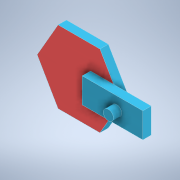
# Autodesk Inventor part: base
Saved by Autodesk Inventor 2021 (Build 250183000, 183)
## iProperties
Created: 2021-08-13
Part Number: base
Material: Genérico
Document SubType Name: Modeling
Designer: uriel
Density: 1 g/cm^3
Appearance: Turquesa
Author: uriel
Autodesk Inventor part; units mm, degrees
ref_plane "YZ Plane" through (0, 0, 0) normal (1, 0, 0) x (0, 1, 0)
ref_plane "XZ Plane" through (0, 0, 0) normal (0, 1, 0) x (-1, 0, 0)
ref_plane "XY Plane" through (0, 0, 0) normal (0, 0, 1) x (1, 0, 0)
sketch "Boceto1" plane through (0, 0, 0) normal (0, 0, 1) x (1, 0, 0)
  line L0 (50, 0) -> (25, -43.3013)
  line L1 (25, -43.3013) -> (-25, -43.3013)
  line L2 (-25, -43.3013) -> (-50, 0)
  line L3 (-50, 0) -> (-25, 43.3013)
  line L4 (-25, 43.3013) -> (25, 43.3013)
  line L5 (25, 43.3013) -> (50, 0)
  point P0 (0, 0)
  point P1 (0, 0)
  dimension "d3" = 50
  constraints: 12 end point, 1 coincident, 13 other
  measures "d3" distance of L4.end L0.start
extrude "Extrusión1" add sketch "Boceto1" along normal blind 10
sketch "Boceto2" plane through (0, 0, 10) normal (0, 0, 1) x (1, 0, 0)
  line L0 (13.773, -15) -> (86.227, -15)
  line L1 (86.227, -15) -> (86.227, 15)
  line L2 (86.227, 15) -> (13.773, 15)
  line L3 (13.773, 15) -> (13.773, -15)
  line L4 (25, -43.3013) -> (50, 0) projected
  line L5 (13.773, -15) -> (86.227, 15) construction
  line L6 (86.227, -15) -> (13.773, 15) construction
  dimension "d7" = 30
  dimension "d8" = 72.454
  constraints: 12 end point, 2 midpoint, 2 parallel, 1 horizontal, 1 perpendicular
  measures "d7" distance of L1.end L0.end
  measures "d8" distance of L1.end L2.end
extrude "Extrusión2" add sketch "Boceto2" along normal blind 10
sketch "Boceto3" plane through (0, 0, 20) normal (0, 0, 1) x (1, 0, 0)
  line L0 (13.773, 15) -> (41.3397, 15) projected
  line L1 (41.3397, 15) -> (25, 43.3013) projected
  line L2 (25, 43.3013) -> (-25, 43.3013) projected
  line L3 (-25, 43.3013) -> (-50, 0) projected
  line L4 (-50, 0) -> (-25, -43.3013) projected
  line L5 (-25, -43.3013) -> (25, -43.3013) projected
  line L6 (25, -43.3013) -> (41.3397, -15) projected
  line L7 (41.3397, -15) -> (13.773, -15) projected
  line L8 (13.773, -15) -> (13.773, 15) projected
  line L9 (0, 0) -> (55, 0)
  circle A0 centre (55, 0) radius 6
  line L10 (13.773, 15) -> (41.3397, 15) projected
  line L11 (41.3397, 15) -> (25, 43.3013) projected
  line L12 (25, 43.3013) -> (-25, 43.3013) projected
  line L13 (-25, 43.3013) -> (-50, 0) projected
  line L14 (-50, 0) -> (-25, -43.3013) projected
  line L15 (-25, -43.3013) -> (25, -43.3013) projected
  line L16 (25, -43.3013) -> (41.3397, -15) projected
  line L17 (41.3397, -15) -> (13.773, -15) projected
  line L18 (13.773, -15) -> (13.773, 15) projected
  line L19 (13.773, 15) -> (41.3397, 15) projected
  line L20 (41.3397, 15) -> (25, 43.3013) projected
  line L21 (25, 43.3013) -> (-25, 43.3013) projected
  line L22 (-25, 43.3013) -> (-50, 0) projected
  line L23 (-50, 0) -> (-25, -43.3013) projected
  line L24 (-25, -43.3013) -> (25, -43.3013) projected
  line L25 (25, -43.3013) -> (41.3397, -15) projected
  line L26 (41.3397, -15) -> (13.773, -15) projected
  line L27 (13.773, -15) -> (13.773, 15) projected
  line L28 (86.227, 15) -> (13.773, 15) projected
  dimension "d9" = 55
  dimension "d10" = 12
  constraints: 2 end point, 1 centre point, 1 coincident, 1 horizontal
  measures "d9" distance of L9.start L9.end
  measures "d10" diameter of A0
extrude "Extrusión3" add sketch "Boceto3" along normal blind 10 contours A0
